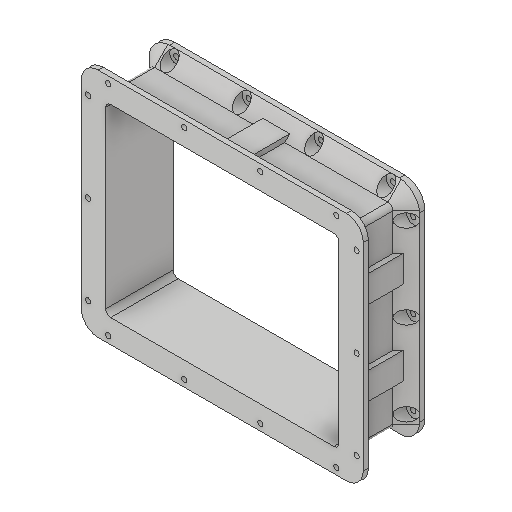
# Autodesk Inventor part: 3DP_PLA_Filter_stage
Saved by Autodesk Inventor 2025 (Build 290162010, 162A)
## iProperties
Created: 2020-03-28
Part Number: 3DP_PLA_Filter_stage
Material: Generic
Document SubType Name: Modeling
Designer: Andrzej
Density: 1 g/cm^3
Appearance: Default
Author: Andrzej
Autodesk Inventor part; units mm, degrees
ref_plane "YZ Plane" through (0, 0, 0) normal (1, 0, 0) x (0, 1, 0)
ref_plane "XZ Plane" through (0, 0, 0) normal (0, 1, 0) x (-1, 0, 0)
ref_plane "XY Plane" through (0, 0, 0) normal (0, 0, 1) x (1, 0, 0)
sketch "Sketch1" plane through (0, 0, 0) normal (0, 0, 1) x (1, 0, 0)
  line L0 (-76, 61) -> (76, 61)
  line L1 (76, 61) -> (76, -61)
  line L2 (76, -61) -> (-76, -61)
  line L3 (-76, -61) -> (-76, 61)
  line L4 (-69.5, 55) -> (69.5, 55)
  line L5 (69.5, 55) -> (69.5, -55)
  line L6 (69.5, -55) -> (-69.5, -55)
  line L7 (-69.5, -55) -> (-69.5, 55)
  line L8 (84, 69) -> (-84, 69)
  line L9 (-84, 69) -> (-84, -69)
  line L10 (-84, -69) -> (84, -69)
  line L11 (84, -69) -> (84, 69)
  line L12 (72.5, 58) -> (-72.5, 58)
  line L13 (-72.5, 58) -> (-72.5, -58)
  line L14 (-72.5, -58) -> (72.5, -58)
  line L15 (72.5, -58) -> (72.5, 58)
  line L16 (0, 109.6961) -> (0, -131.8013)
  line L17 (-145.0248, 0) -> (154.2595, 0)
  point P0 (0, 0)
  point P1 (-68, -65)
  point P2 (-80, -53)
  point P3 (-22.6667, -65)
  point P4 (22.6667, -65)
  point P5 (68, -65)
  point P6 (-80, 0)
  point P7 (-80, 53)
  point P8 (80, -53)
  point P9 (80, 0)
  point P10 (80, 53)
  point P11 (-68, 65)
  point P12 (-22.6667, 65)
  point P13 (22.6667, 65)
  point P14 (68, 65)
  dimension "d0" = 152
  dimension "d1" = 122
  dimension "d2" = 139
  dimension "d3" = 110
  dimension "d4" = 6
  dimension "d5" = 6.5
  dimension "d6" = 8
  dimension "d7" = 3
  dimension "d44" = 69.5
  dimension "d45" = 55
  dimension "d84" = 4
  dimension "d85" = 4
  dimension "d87" = 16
  dimension "d88" = 16
  dimension "d89" = 168
  dimension "d90" = 138
  dimension "d93" = 45.3333
  dimension "d100" = 53
  constraints: 36 end point, 8 parallel, 7 symmetric about line, 4 horizontal, 4 perpendicular, 2 vertical, 11 other
  measures "d0" distance of L1.end L2.end
  measures "d1" distance of L0.end L1.end
  measures "d2" distance of L5.end L6.end
  measures "d3" distance of L4.end L5.end
  measures "d4" distance between parallel lines of L0 L4
  measures "d5" distance between parallel lines of L3 L7
  measures "d6" distance between parallel lines of L0 L8
  measures "d7" distance between parallel lines of L4 L12
  measures "d44" distance from line of point (0, 0) L5
  measures "d45" distance from line of point (0, 0) L6
  measures "d84" distance from line of L2 point (-68, -65)
  measures "d85" distance from line of L3 point (-80, -53)
  measures "d87" distance from line of L9 point (-68, -65)
  measures "d88" distance from line of point (-80, -53) L10
  measures "d89" distance between parallel lines of L11 L9
  measures "d90" distance of L8.end L9.end
  measures "d93" distance of point (-68, -65) point (-22.667, -65)
  measures "d100" distance of point (-80, -53) point (-80, 0)
extrude "Extrusion1" add sketch "Sketch1" along normal blind 3 contours L3 L17 L9 L8 L16 L0 | L0 L16 L12 L13 L17 L3 | L16 L8 L11 L17 L1 L0 | L0 L1 L17 L15 L12 L16 | L17 L13 L14 L16 L2 L3 | L3 L2 L16 L10 L9 L17 | L16 L4 L7 L17 L13 L12 | L12 L15 L17 L5 L4 L16 | L17 L7 L6 L16 L14 L13 | L17 L11 L10 L16 L2 L1 | L1 L2 L16 L14 L15 L17 | L15 L14 L16 L6 L5 L17
extrude "Extrusion2" add sketch "Sketch1" against normal blind 34.2 contours L16 L4 L7 L17 L13 L12 | L12 L15 L17 L5 L4 L16 | L17 L7 L6 L16 L14 L13 | L15 L14 L16 L6 L5 L17
sketch "Sketch2" plane through (0, 0, -34.2) normal (0, 0, -1) x (-1, 0, 0)
  line L0 (69.5, 55) -> (69.5, -55) projected
  line L1 (69.5, -55) -> (-69.5, -55) projected
  line L2 (-69.5, -55) -> (-69.5, 55) projected
  line L3 (-69.5, 55) -> (69.5, 55) projected
  line L4 (72.5, 58) -> (-72.5, 58) projected
  line L5 (-72.5, 58) -> (-72.5, -58) projected
  line L6 (-72.5, -58) -> (72.5, -58) projected
  line L7 (72.5, -58) -> (72.5, 58) projected
  line L8 (-80.5, 66) -> (80.5, 66)
  line L9 (80.5, 66) -> (80.5, -66)
  line L10 (80.5, -66) -> (-80.5, -66)
  line L11 (-80.5, -66) -> (-80.5, 66)
  point P0 (0, 0)
  dimension "d15" = 8
  constraints: 8 end point, 3 other
  measures "d15" distance between parallel lines of L4 L8
extrude "Extrusion3" add sketch "Sketch2" along normal blind 3 contours L7 L6 L5 L4 | L8 L9 L10 L11
fillet "Fillet5" radius 3 8 edges at (72.5, 58, -17.1) (69.5, 55, -17.1) (-72.5, 58, -17.1) (-69.5, 55, -17.1) (-69.5, -55, -17.1) (-72.5, -58, -17.1) (72.5, -58, -17.1) (69.5, -55, -17.1)
chamfer "Chamfer1" distance 8 angle 45 8 edges at (72.5, 0, -34.2) (71.6213, -57.1213, -34.2) (0, -58, -34.2) (-71.6213, -57.1213, -34.2) (-72.5, 0, -34.2) (-71.6213, 57.1213, -34.2) (0, 58, -34.2) (71.6213, 57.1213, -34.2)
fillet "Fillet6" radius 8 8 edges at (71.6213, 57.1213, 0) (0, 58, 0) (-71.6213, 57.1213, 0) (-72.5, 0, 0) (-71.6213, -57.1213, 0) (0, -58, 0) (71.6213, -57.1213, 0) (72.5, 0, 0)
sketch "Sketch3" plane through (0, 0, -37.2) normal (0, 0, -1) x (-1, 0, 0)
  line L0 (66.5, -55) -> (-66.5, -55) projected
  arc A0 (-69.5, -52) -> (-66.5, -55) centre (-66.5, -52) ccw projected
  line L1 (-69.5, -52) -> (-69.5, 52) projected
  arc A1 (-66.5, 55) -> (-69.5, 52) centre (-66.5, 52) ccw projected
  line L2 (-66.5, 55) -> (66.5, 55) projected
  arc A2 (69.5, 52) -> (66.5, 55) centre (66.5, 52) ccw projected
  line L3 (69.5, 52) -> (69.5, -52) projected
  arc A3 (66.5, -55) -> (69.5, -52) centre (66.5, -52) ccw projected
  line L4 (80.5, 66) -> (-80.5, 66) projected
  line L5 (-80.5, 66) -> (-80.5, -66) projected
  line L6 (-80.5, -66) -> (80.5, -66) projected
  line L7 (80.5, -66) -> (80.5, 66) projected
  line L8 (-72.5, 55) -> (-72.5, -55) projected
  arc A4 (-72.5, -55) -> (-69.5, -58) centre (-69.5, -55) ccw projected
  line L9 (-69.5, -58) -> (69.5, -58) projected
  arc A5 (69.5, -58) -> (72.5, -55) centre (69.5, -55) ccw projected
  line L10 (72.5, -55) -> (72.5, 55) projected
  arc A6 (72.5, 55) -> (69.5, 58) centre (69.5, 55) ccw projected
  line L11 (69.5, 58) -> (-69.5, 58) projected
  arc A7 (-69.5, 58) -> (-72.5, 55) centre (-69.5, 55) ccw projected
  line L12 (0, 81.075) -> (0, -86.5842)
  line L13 (-130.8744, 0) -> (120.838, 0)
  point P0 (0, 0)
  point P1 (-64.5, -62)
  point P2 (-76.5, -50)
  point P3 (-21.5, -62)
  point P4 (21.5, -62)
  point P5 (64.5, -62)
  point P6 (-76.5, 0)
  point P7 (-76.5, 50)
  point P8 (76.5, -50)
  point P9 (76.5, 0)
  point P10 (76.5, 50)
  point P11 (-64.5, 62)
  point P12 (-21.5, 62)
  point P13 (21.5, 62)
  point P14 (64.5, 62)
  dimension "d24" = 8
  dimension "d25" = 4
  dimension "d26" = 16
  dimension "d27" = 161
  dimension "d28" = 132
  dimension "d29" = 16
  dimension "d32" = 43
  dimension "d39" = 50
  dimension "d70" = 4
  constraints: 7 symmetric about line, 4 end point, 2 horizontal, 2 vertical, 5 other
  measures "d24" distance between parallel lines of L6 L9
  measures "d25" distance from line of L6 point (-64.5, -62)
  measures "d26" distance from line of L5 point (-64.5, -62)
  measures "d27" distance between parallel lines of L5 L7
  measures "d28" distance of L4.end L5.end
  measures "d29" distance from line of L6 point (-76.5, -50)
  measures "d32" distance of point (-64.5, -62) point (-21.5, -62)
  measures "d39" distance of point (-76.5, -50) point (-76.5, 0)
  measures "d70" distance from line of L5 point (-76.5, -50)
hole "Hole1" at (64.5, -62, -37.2) at (76.5, -50, -37.2) at (21.5, -62, -37.2) at (-21.5, -62, -37.2) at (-64.5, -62, -37.2) at (76.5, 0, -37.2) at (76.5, 50, -37.2) at (-76.5, 50, -37.2) at (-76.5, 0, -37.2) at (-76.5, -50, -37.2) at (64.5, 62, -37.2) at (21.5, 62, -37.2) at (-21.5, 62, -37.2) at (-64.5, 62, -37.2) direction (0, 0, 1) diameter 3.2 depth 15 tip angle 118
sketch "Sketch4" plane through (0, 0, -34.2) normal (0, 0, 1) x (1, 0, 0)
  circle A0 centre (-21.5, 62) radius 1.6 projected
  circle A1 centre (64.5, 62) radius 1.6 projected
  circle A2 centre (-76.5, 0) radius 1.6 projected
  circle A3 centre (76.5, 50) radius 1.6 projected
  circle A4 centre (-64.5, -62) radius 1.6 projected
  circle A5 centre (21.5, -62) radius 1.6 projected
  circle A6 centre (64.5, -62) radius 1.6 projected
  circle A7 centre (76.5, -50) radius 1.6 projected
  circle A8 centre (-21.5, -62) radius 1.6 projected
  circle A9 centre (76.5, 0) radius 1.6 projected
  circle A10 centre (-76.5, 50) radius 1.6 projected
  circle A11 centre (-76.5, -50) radius 1.6 projected
  circle A12 centre (21.5, 62) radius 1.6 projected
  circle A13 centre (-64.5, 62) radius 1.6 projected
  line L0 (-66.5, -55) -> (66.5, -55) projected
  arc A14 (66.5, -55) -> (69.5, -52) centre (66.5, -52) ccw projected
  line L1 (69.5, -52) -> (69.5, 52) projected
  arc A15 (69.5, 52) -> (66.5, 55) centre (66.5, 52) ccw projected
  line L2 (66.5, 55) -> (-66.5, 55) projected
  arc A16 (-66.5, 55) -> (-69.5, 52) centre (-66.5, 52) ccw projected
  line L3 (-69.5, 52) -> (-69.5, -52) projected
  arc A17 (-69.5, -52) -> (-66.5, -55) centre (-66.5, -52) ccw projected
  line L4 (-80.5, 66) -> (80.5, 66) projected
  line L5 (80.5, 66) -> (80.5, -66) projected
  line L6 (80.5, -66) -> (-80.5, -66) projected
  line L7 (-80.5, -66) -> (-80.5, 66) projected
  circle A18 centre (-64.5, 62) radius 4
  circle A19 centre (-21.5, 62) radius 4
  circle A20 centre (21.5, 62) radius 4
  circle A21 centre (64.5, 62) radius 4
  circle A22 centre (76.5, 50) radius 4
  circle A23 centre (76.5, 0) radius 4
  circle A24 centre (76.5, -50) radius 4
  circle A25 centre (64.5, -62) radius 4
  circle A26 centre (21.5, -62) radius 4
  circle A27 centre (-21.5, -62) radius 4
  circle A28 centre (-64.5, -62) radius 4
  circle A29 centre (-76.5, -50) radius 4
  circle A30 centre (-76.5, 0) radius 4
  circle A31 centre (-76.5, 50) radius 4
  line L8 (-69.5, -58) -> (69.5, -58) projected
  line L9 (69.5, -58) -> (-69.5, -58) projected
  line L10 (72.5, -55) -> (72.5, 55) projected
  line L11 (72.5, 55) -> (72.5, -55) projected
  line L12 (69.5, 58) -> (-69.5, 58) projected
  line L13 (-69.5, 58) -> (69.5, 58) projected
  line L14 (-72.5, 55) -> (-72.5, -55) projected
  line L15 (-72.5, -55) -> (-72.5, 55) projected
  line L16 (-8, -58) -> (8, -58)
  line L17 (8, -58) -> (8, -61)
  line L18 (8, -61) -> (-8, -61)
  line L19 (-8, -61) -> (-8, -58)
  line L20 (-106.8891, 0) -> (109.3807, 0)
  line L21 (0, 87.8366) -> (0, -109.5258)
  line L22 (-72.5, 33) -> (-75.5, 33)
  line L23 (-75.5, 33) -> (-75.5, 17)
  line L24 (-75.5, 17) -> (-72.5, 17)
  line L25 (-72.5, 17) -> (-72.5, 33)
  line L26 (-72.5, -17) -> (-75.5, -17)
  line L27 (-75.5, -17) -> (-75.5, -33)
  line L28 (-75.5, -33) -> (-72.5, -33)
  line L29 (-72.5, -33) -> (-72.5, -17)
  line L30 (72.5, 33) -> (75.5, 33)
  line L31 (75.5, 33) -> (75.5, 17)
  line L32 (75.5, 17) -> (72.5, 17)
  line L33 (72.5, 17) -> (72.5, 33)
  line L34 (72.5, -17) -> (75.5, -17)
  line L35 (75.5, -17) -> (75.5, -33)
  line L36 (75.5, -33) -> (72.5, -33)
  line L37 (72.5, -33) -> (72.5, -17)
  line L38 (-8, 58) -> (8, 58)
  line L39 (8, 58) -> (8, 61)
  line L40 (8, 61) -> (-8, 61)
  line L41 (-8, 61) -> (-8, 58)
  point P0 (0, 0)
  dimension "d53" = 8
  dimension "d54" = 8
  dimension "d55" = 8
  dimension "d56" = 8
  dimension "d57" = 8
  dimension "d58" = 8
  dimension "d59" = 8
  dimension "d60" = 8
  dimension "d61" = 8
  dimension "d62" = 8
  dimension "d63" = 8
  dimension "d64" = 8
  dimension "d65" = 8
  dimension "d66" = 8
  dimension "d71" = 16
  dimension "d72" = 3
  dimension "d73" = 8
  dimension "d74" = 3
  dimension "d75" = 16
  dimension "d76" = 3
  dimension "d77" = 16
  dimension "d78" = 50
  dimension "d79" = 17
  dimension "d80" = 17
  constraints: 52 end point, 14 centre point, 14 coincident, 12 symmetric about line, 6 parallel, 4 horizontal, 3 perpendicular, 3 point on line, 1 vertical
  measures "d53" diameter of A18
  measures "d54" diameter of A19
  measures "d55" diameter of A20
  measures "d56" diameter of A21
  measures "d57" diameter of A22
  measures "d58" diameter of A23
  measures "d59" diameter of A24
  measures "d60" diameter of A25
  measures "d61" diameter of A26
  measures "d62" diameter of A27
  measures "d63" diameter of A28
  measures "d64" diameter of A29
  measures "d65" diameter of A30
  measures "d66" diameter of A31
  measures "d71" distance of L17.end L18.end
  measures "d72" distance of L16.end L17.end
  measures "d73" distance from line of point (0, 0) L19
  measures "d74" distance of L24.end L23.end
  measures "d75" distance of L23.end L22.end
  measures "d76" distance of L28.end L27.end
  measures "d77" distance of L27.end L26.end
  measures "d78" distance of A11.centre A2.centre
  measures "d79" distance from line of L26 A2.centre
  measures "d80" distance from line of A2.centre L24
extrude "Extrusion4" cut sketch "Sketch4" along normal blind 10 contours L20 A30 A2 | A2 L20 A30 | A29 | A31 | A28 | A18 | L20 A9 A23 | A23 L20 A9 | A27 | A19 | A22 | A24 | A20 | A26 | A21 | A25
fillet "Fillet7" radius 12 4 edges at (80.5, 66, -35.7) (-80.5, 66, -35.7) (-80.5, -66, -35.7) (80.5, -66, -35.7)
extrude "Extrusion5" add sketch "Sketch4" along normal up to surface (34.2 mm away) contours L24 L23 L22 L14 | L14 L28 L27 L26 | L21 L40 L39 L12 | L12 L41 L40 L21 | L21 L18 L19 L8 | L8 L17 L18 L21 | L34 L35 L36 L10 | L10 L30 L31 L32
fillet "Fillet8" radius 10 4 edges at (-84, -69, 1.5) (84, -69, 1.5) (84, 69, 1.5) (-84, 69, 1.5)
hole "Hole2" at (-68, -65, 0) at (-80, -53, 0) at (-22.6667, -65, 0) at (22.6667, -65, 0) at (68, -65, 0) at (-80, 0, 0) at (-80, 53, 0) at (80, 53, 0) at (80, 0, 0) at (80, -53, 0) at (-68, 65, 0) at (-22.6667, 65, 0) at (22.6667, 65, 0) at (68, 65, 0) direction (0, 0, 1) diameter 3.2 depth 3 tip angle 118
hole "Hole3" at (68, 65, 0) at (22.6667, 65, 0) at (-22.6667, 65, 0) at (-68, 65, 0) at (-80, 53, 0) at (-80, 0, 0) at (-80, -53, 0) at (-68, -65, 0) at (-22.6667, -65, 0) at (22.6667, -65, 0) at (68, -65, 0) at (80, -53, 0) at (80, 0, 0) at (80, 53, 0) direction (0, 0, -1) diameter 8 depth 5 tip angle 118
equation "\"d4\" = -0.5 * d3 + 0.5 * d1"
equation "\"d5\" = -0.5 * d2 + 0.5 * d0"
equation "\"d44\" = 0.5 * d2"
equation "\"d45\" = 0.5 * d3"
equation "\"d84\" = 0.5 * d6"
equation "\"d85\" = d84"
equation "\"d88\" = d87"
equation "\"d93\" = -0.666667 * d87 + 0.333333 * d89"
equation "\"d100\" = -d88 + 0.5 * d90"
equation "\"d25\" = 0.5 * d24"
equation "\"d29\" = d26"
equation "\"d32\" = -0.666667 * d26 + 0.333333 * d27"
equation "\"d39\" = -d29 + 0.5 * d28"
equation "\"d70\" = d25"
equation "\"d73\" = 0.5 * d71"
equation "\"d79\" = -0.5 * d77 + 0.5 * d78"
equation "\"d80\" = d79"
body "Solid1"
